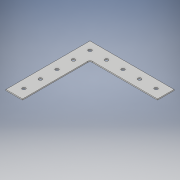
# Autodesk Inventor part: Gusset 2B 2.0
Saved by Autodesk Inventor 2018 (Build 220112000, 112)
## iProperties
Created: 2017-10-12
Part Number: Gusset 2B 2.0
Material: Generic
Document SubType Name: Modeling
Designer: s-2512711
Density: 1 g/cm^3
Appearance: Default
Author: s-2512711
Autodesk Inventor part; units mm, degrees
ref_plane "YZ Plane" through (0, 0, 0) normal (1, 0, 0) x (0, 1, 0)
ref_plane "XZ Plane" through (0, 0, 0) normal (0, 1, 0) x (-1, 0, 0)
ref_plane "XY Plane" through (0, 0, 0) normal (0, 0, 1) x (1, 0, 0)
sketch "Sketch1" plane through (0, 0, 0) normal (0, 1, 0) x (-1, 0, 0)
  line L0 (0, 0) -> (-25.4, 0)
  line L1 (-25.4, -35.921) -> (-25.4, -127)
  line L2 (-25.4, -152.4) -> (0, -152.4)
  line L3 (0, -152.4) -> (0, 0)
  line L4 (0, -152.4) -> (-152.4, -152.4)
  line L5 (-152.4, -152.4) -> (-152.4, -127)
  line L6 (-116.479, -127) -> (-25.4, -127)
  line L7 (0, -127) -> (0, -152.4)
  line L8 (-152.4, -127) -> (-25.4, 0)
  line L9 (-25.4, -35.921) -> (-116.479, -127)
  dimension "d0" = 25.4
  dimension "d1" = 152.4
  dimension "d2" = 152.4
  dimension "d3" = 25.4
  dimension "d4" = 25.4
  constraints: 20 end point, 5 parallel, 2 horizontal, 2 perpendicular
  measures "d0" distance of L2.end L2.start
  measures "d1" distance of L0.end L2.start
  measures "d2" distance of L5.end L7.start
  measures "d3" distance of L4.end L5.end
  measures "d4" distance between parallel lines of L8 L9
extrude "Extrusion1" add sketch "Sketch1" along normal blind 1.5875
sketch "Sketch2" plane through (0, 1.5875, 0) normal (0, 1, 0) x (1, 0, 0)
  line L0 (152.4, 152.4) -> (0, 152.4) projected
  line L1 (0, 152.4) -> (25.4, 152.4)
  line L2 (25.4, 35.921) -> (25.4, 127) projected
  line L3 (25.4, 152.4) -> (25.4, 127)
  line L4 (25.4, 127) -> (0, 152.4)
  line L5 (25.4, 152.4) -> (0, 127)
  line L6 (0, 152.4) -> (0, 0) projected
  line L7 (12.7, 139.7) -> (38.1, 139.7)
  line L8 (38.1, 139.7) -> (63.5, 139.7)
  line L9 (63.5, 139.7) -> (88.9, 139.7)
  line L10 (88.9, 139.7) -> (114.3, 139.7)
  line L11 (114.3, 139.7) -> (139.7, 139.7)
  line L12 (12.7, 139.7) -> (12.7, 114.3)
  line L13 (12.7, 114.3) -> (12.7, 88.9)
  line L14 (12.7, 88.9) -> (12.7, 63.5)
  line L15 (12.7, 63.5) -> (12.7, 38.1)
  line L16 (12.7, 38.1) -> (12.7, 12.7)
  circle A0 centre (12.7, 139.7) radius 2.54
  circle A1 centre (38.1, 139.7) radius 2.54
  circle A2 centre (63.5, 139.7) radius 2.54
  circle A3 centre (88.9, 139.7) radius 2.54
  circle A4 centre (114.3, 139.7) radius 2.54
  circle A5 centre (139.7, 139.7) radius 2.54
  circle A6 centre (12.7, 114.3) radius 2.54
  circle A7 centre (12.7, 88.9) radius 2.54
  circle A8 centre (12.7, 63.5) radius 2.54
  circle A9 centre (12.7, 38.1) radius 2.54
  circle A10 centre (12.7, 12.7) radius 2.54
  dimension "d7" = 25.4
  dimension "d8" = 25.4
  dimension "d9" = 25.4
  dimension "d10" = 25.4
  dimension "d11" = 25.4
  dimension "d12" = 25.4
  dimension "d13" = 25.4
  dimension "d14" = 25.4
  dimension "d15" = 25.4
  dimension "d16" = 25.4
  dimension "d17" = 5.08
  dimension "d18" = 5.08
  dimension "d19" = 5.08
  dimension "d20" = 5.08
  dimension "d21" = 5.08
  dimension "d22" = 5.08
  dimension "d23" = 5.08
  dimension "d24" = 5.08
  constraints: 28 end point, 11 centre point, 11 coincident, 10 point on line, 1 horizontal, 1 midpoint, 1 perpendicular, 1 vertical
  measures "d7" distance of L0.end L1.end
  measures "d8" distance of L7.end L8.end
  measures "d9" distance of L8.end L9.end
  measures "d10" distance of L9.end L10.end
  measures "d11" distance of L10.end L11.end
  measures "d12" distance of L7.start L12.end
  measures "d13" distance of L12.end L13.end
  measures "d14" distance of L13.end L14.end
  measures "d15" distance of L14.end L15.end
  measures "d16" distance of L15.end L16.end
  measures "d17" diameter of A0
  measures "d18" diameter of A1
  measures "d19" diameter of A2
  measures "d20" diameter of A3
  measures "d21" diameter of A4
  measures "d22" diameter of A5
  measures "d23" diameter of A6
  measures "d24" diameter of A7
hole "Hole1" at (12.7, 1.5875, -139.7) at (38.1, 1.5875, -139.7) at (63.5, 1.5875, -139.7) at (88.9, 1.5875, -139.7) at (114.3, 1.5875, -139.7) at (12.7, 1.5875, -114.3) at (12.7, 1.5875, -88.9) at (12.7, 1.5875, -63.5) at (12.7, 1.5875, -38.1) direction (0, -1, 0) diameter 5.08 end through all
sketch "Sketch3" plane through (0, 1.5875, 0) normal (0, 1, 0) x (1, 0, 0)
  line L0 (116.479, 127) -> (25.4, 127) projected
  line L1 (116.479, 127) -> (129.179, 127)
  line L2 (129.179, 127) -> (129.179, 152.4)
  line L3 (152.4, 152.4) -> (0, 152.4) projected
  line L4 (25.4, 35.921) -> (25.4, 127) projected
  line L5 (25.4, 35.921) -> (25.4, 23.221)
  line L6 (25.4, 23.221) -> (0, 23.221)
  line L7 (0, 23.221) -> (0, 0)
  line L8 (25.4, 0) -> (152.4, 127) projected
  line L9 (0, 0) -> (25.4, 0)
  line L10 (25.4, 0) -> (152.4, 127)
  line L11 (152.4, 127) -> (152.4, 152.4) projected
  line L12 (152.4, 127) -> (152.4, 152.4)
  line L13 (152.4, 152.4) -> (129.179, 152.4)
  line L14 (116.479, 127) -> (25.4, 35.921)
  dimension "d32" = 12.7
  dimension "d33" = 12.7
  constraints: 20 end point, 5 perpendicular, 2 parallel, 1 collinear, 1 horizontal, 1 point on line, 1 vertical
  measures "d32" distance of L0.start L1.end
  measures "d33" distance of L4.start L5.end
extrude "Extrusion2" cut sketch "Sketch3" against normal blind 1.5875 contours L1 L2 L3 L11 L8 L9 L7 L6 L5 L14
sketch "Sketch4" plane through (0, 1.5875, 0) normal (0, 1, 0) x (1, 0, 0)
  line L0 (129.179, 127) -> (25.4, 127) projected
  line L1 (129.179, 127) -> (25.4, 23.221)
  line L2 (25.4, 59.142) -> (93.258, 127)
  line L3 (25.4, 127) -> (25.4, 23.221) projected
  line L4 (25.4, 59.142) -> (25.4, 23.221)
  point P0 (0, 0)
  dimension "d36" = 25.4
  constraints: 6 end point, 1 coincident, 1 collinear, 1 point on line
  measures "d36" distance between parallel lines of L1 L2
extrude "Extrusion3" add sketch "Sketch4" against normal blind 1.5875 contours L1 L3 L2 L0
fillet "Fillet1" radius 3.175 3 edges at (25.4, 0.7937, -127) (93.258, 0.7937, -127) (25.4, 0.7937, -59.142)
sketch "Sketch5" plane through (0, 1.5875, 0) normal (0, 1, 0) x (1, 0, 0)
  line L0 (25.4, 123.825) -> (25.4, 66.8072) projected
  line L1 (25.4, 23.221) -> (25.4, 123.825)
  line L2 (85.5928, 127) -> (28.575, 127) projected
  line L3 (28.575, 127) -> (135.0414, 127)
  line L4 (135.0414, 127) -> (135.0414, 23.221)
  line L5 (135.0414, 23.221) -> (25.4, 23.221)
  line L6 (28.575, 127) -> (85.5928, 127) projected
  line L7 (28.575, 127) -> (25.4, 123.825)
  point P0 (0, 0)
  constraints: 10 end point, 2 collinear, 2 perpendicular
extrude "Extrusion4" cut sketch "Sketch5" against normal blind 25.4
body "Solid1"
